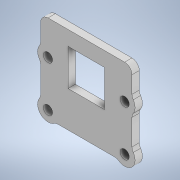
# Autodesk Inventor part: CameraFilterPlate
Saved by Autodesk Inventor 2020 (Build 240168000, 168)
## iProperties
Created: 2019-04-29
Part Number: CameraFilterPlate
Material: Generic
Document SubType Name: Modeling
Designer: Connor
Density: 1 g/cm^3
Appearance: Default
Author: Connor
Autodesk Inventor part; units mm, degrees
ref_plane "YZ Plane" through (0, 0, 0) normal (1, 0, 0) x (0, 1, 0)
ref_plane "XZ Plane" through (0, 0, 0) normal (0, 1, 0) x (-1, 0, 0)
ref_plane "XY Plane" through (0, 0, 0) normal (0, 0, 1) x (1, 0, 0)
sketch "Sketch1" plane through (0, 0, 0) normal (0, 0, 1) x (1, 0, 0)
  line L0 (0, 0) -> (25, 0)
  line L1 (25, 0) -> (25, 23.862)
  line L2 (25, 23.862) -> (0, 23.862)
  line L3 (0, 23.862) -> (0, 0)
  circle A0 centre (2, 2) radius 1.25
  circle A1 centre (23, 2) radius 1.25
  circle A2 centre (2, 14.5) radius 1.25
  circle A3 centre (23, 14.5) radius 1.25
  line L4 (7.5, 19.862) -> (17.5, 19.862)
  line L5 (17.5, 19.862) -> (17.5, 9.862)
  line L6 (17.5, 9.862) -> (7.5, 9.862)
  line L7 (7.5, 9.862) -> (7.5, 19.862)
  line L8 (0, 23.862) -> (7.5, 19.862) construction
  line L9 (17.5, 19.862) -> (25, 23.862) construction
  dimension "d0" = 25
  dimension "d1" = 23.862
  dimension "d2" = 2.5
  dimension "d3" = 2
  dimension "d4" = 2
  dimension "d5" = 14.5
  dimension "d6" = 2
  dimension "d7" = 10
  dimension "d8" = 4
  constraints: 20 end point, 4 centre point, 4 parallel, 3 equal radius, 2 equal length, 2 horizontal, 2 horizontal alignment, 2 perpendicular, 2 vertical alignment
  measures "d0" distance of L1.end L2.end
  measures "d1" distance of L0.end L1.end
  measures "d2" diameter of A0
  measures "d3" distance from line of L3 A0.centre
  measures "d4" distance from line of L0 A0.centre
  measures "d5" distance from line of L0 A3.centre
  measures "d6" distance from line of L1 A1.centre
  measures "d7" distance of L4.start L4.end
  measures "d8" distance between parallel lines of L2 L4
extrude "Extrusion1" add sketch "Sketch1" along normal blind 2
fillet "Fillet1" radius 2 4 edges at (25, 23.862, 1) (0, 23.862, 1) (0, 0, 1) (25, 0, 1)
sketch "Sketch2" plane through (0, 0, 2) normal (0, 0, 1) x (1, 0, 0)
  circle A0 centre (2, 14.5) radius 1.25 projected
  circle A1 centre (2, 2) radius 1.25 projected
  circle A2 centre (23, 2) radius 1.25 projected
  circle A3 centre (23, 14.5) radius 1.25 projected
  circle A4 centre (2, 14.5) radius 2.85
  circle A5 centre (2, 2) radius 2.85
  circle A6 centre (23, 2) radius 2.85
  circle A7 centre (23, 14.5) radius 2.85
  point P0 (0, 0)
  dimension "d12" = 1.6
  constraints: 4 centre point, 3 equal radius
  measures "d12" radial gap between concentric circles of A0 A4
extrude "Extrusion2" add sketch "Sketch2" against normal up to surface (2 mm away)
fillet "Fillet2" radius 2 8 edges at (0, 16.5304, 1) (0, 12.4696, 1) (0, 4.0304, 1) (4.0304, 0, 1) (20.9696, 0, 1) (25, 4.0304, 1) (25, 16.5304, 1) (25, 12.4696, 1)
body "Solid1"
